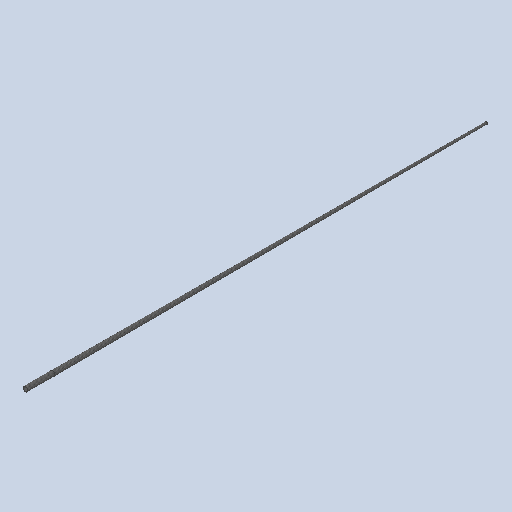
# Autodesk Inventor part: False Rear Spar Final
Saved by Autodesk Inventor 2025.2 (Build 292293000, 293)
## iProperties
Created: 2024-12-29
Part Number: False Rear Spar Final
Material: CFRP
Document SubType Name: Modeling
Designer: hjbre
Density: 1.43 g/cm^3
Appearance: Carbon Fiber
Author: hjbre
Autodesk Inventor part; units mm, degrees
ref_plane "YZ Plane" through (0, 0, 0) normal (1, 0, 0) x (0, 1, 0)
ref_plane "XZ Plane" through (0, 0, 0) normal (0, 1, 0) x (-1, 0, 0)
ref_plane "XY Plane" through (0, 0, 0) normal (0, 0, 1) x (1, 0, 0)
sketch "Sketch1" plane through (0, 0, 0) normal (1, 0, 0) x (0, 1, 0)
  point P0 (0, 0)
sketch "Sketch2" plane through (0, 0, 0) normal (1, 0, 0) x (0, 1, 0)
  line L0 (0, 0) -> (6.77, 0)
  line L1 (0, 0) -> (0, -1200)
  line L2 (0, -1200) -> (3.1, -1200)
  line L3 (3.1, -1200) -> (6.77, 0)
  line L4 (0, 0) -> (0, 75)
  line L5 (0, 75) -> (6.77, 75)
  line L6 (6.77, 75) -> (6.77, 0)
  dimension "d0" = 6.77
  dimension "d1" = 1200
  dimension "d2" = 3.1
  dimension "d5" = 75
  constraints: 14 end point, 3 perpendicular, 2 vertical, 1 horizontal
  measures "d0" distance of L0.start L0.end
  measures "d1" distance of L0.start L1.end
  measures "d2" distance of L1.end L2.end
  measures "d5" distance of L0.start L4.end
revolve "Revolution1" add sketch "Sketch2" angle 360 about axis through (0, 0, 0) along (0, 0, -1)
shell "Shell1" thickness 1 removed faces 1 at (1.6044, -0.8002, 75)
body "Solid1"
